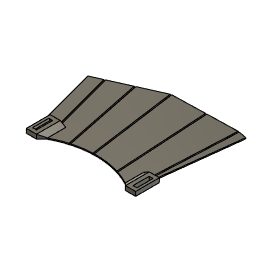
Base-plate (Autodesk Fusion 360 design; units mm, degrees)
Autodesk Fusion 360 part; units mm, degrees
sketch "Sketch1" plane through (0, 0, 0) normal (0, 1, 0) x (1, 0, 0)
  line L0 (-33, 0) -> (52, 0)
  line L1 (-33, 0) -> (-44.6469, 43.4667)
  line L2 (-35.3975, 47.5847) -> (-22.6472, 0)
  line L3 (-18.9537, 54.906) -> (-7.6472, 0)
  line L4 (52, 0) -> (59.5264, 63.5559)
  line L5 (31.5, 0) -> (27.6688, 64.3091)
  line L6 (47.3528, 0) -> (47.3528, -15)
  line L7 (47.3528, -15) -> (-22.6472, -15)
  line L8 (-22.6472, -15) -> (-22.6472, 0)
  line L9 (50.3528, -3.25) -> (52.3528, -3.25)
  line L10 (52.3528, -3.25) -> (52.3528, -15.95)
  line L11 (52.3528, -15.95) -> (50.3528, -15.95)
  line L12 (50.3528, -15.95) -> (50.3528, -3.25)
  line L13 (-27.6472, -3.25) -> (-25.6472, -3.25)
  line L14 (-25.6472, -3.25) -> (-25.6472, -15.95)
  line L15 (-25.6472, -15.95) -> (-27.6472, -15.95)
  line L16 (-27.6472, -15.95) -> (-27.6472, -3.25)
  line L17 (-22.6472, -0.25) -> (-30.6472, -0.25)
  line L18 (-30.6472, -0.25) -> (-30.6472, -18.95)
  line L19 (-30.6472, -18.95) -> (-22.6472, -18.95)
  line L20 (-22.6472, -18.95) -> (-22.6472, -15)
  line L21 (47.3528, -15) -> (47.3528, -18.95)
  line L22 (47.3528, -18.95) -> (55.3528, -18.95)
  line L23 (55.3528, -18.95) -> (55.3528, -0.25)
  line L24 (55.3528, -0.25) -> (47.3528, -0.25)
  line L25 (0.6769, 63.6461) -> (9.5, 0)
  line L26 (49.5, 0) -> (52.6612, 64.9231)
  line L27 (12.3528, -15) -> (10.1055, -68.0076)
  arc A0 (43.4028, -15) -> (-18.6972, -15) centre (12.3528, -72.1043) ccw
  line L28 (-44.6469, 43.4667) -> (-35.3975, 47.5847)
  line L29 (-35.3975, 47.5847) -> (-18.9537, 54.906)
  line L30 (-18.9537, 54.906) -> (0.6769, 63.6461)
  line L31 (0.6769, 63.6461) -> (27.6688, 64.3091)
  line L32 (27.6688, 64.3091) -> (52.6612, 64.9231)
  line L33 (59.5264, 63.5559) -> (52.6612, 64.9231)
  dimension "d1" = 85
  dimension "d2" = 33
  dimension "d4" = 105
  dimension "d5" = 45
  dimension "d12" = 10
  dimension "d15" = 18
  dimension "d19" = 37.5
  dimension "d22" = 7
  dimension "d29" = 15
  dimension "d30" = 2
  dimension "d31" = 12.7
  dimension "d32" = 2
  dimension "d33" = 12.7
  dimension "d34" = 3.25
  dimension "d35" = 3.25
  dimension "d36" = 3
  dimension "d37" = 3
  dimension "d38" = 3
  dimension "d39" = 3
  dimension "d40" = 3
  dimension "d41" = 3
  dimension "d42" = 3
  dimension "d43" = 3
  dimension "d45" = 64
  dimension "d96" = 70
  dimension "d98" = 7
  dimension "d101" = 15
  dimension "d102" = 22
  dimension "d115" = 3.95
  dimension "d116" = 3.95
  dimension "d117" = 21.4884
  dimension "d120" = 27
  dimension "d121" = 25
  dimension "d123" = 99
  dimension "d124" = 18
  dimension "d125" = 65
  dimension "d127" = 65
  constraint coincident L0 L2.end
  constraint parallel L1 L2
  constraint coincident L0 L3.end
  constraint coincident L0 L6.start
  constraint coincident L0 L5.start
  constraint horizontal L0
  constraint perpendicular L0 L6
  constraint perpendicular L6 L7
  constraint perpendicular L0 L8
  constraint horizontal L9
  constraint vertical L10
  constraint horizontal L11
  constraint vertical L12
  constraint horizontal L13
  constraint vertical L14
  constraint horizontal L15
  constraint vertical L16
  constraint coincident L8 L17.start
  constraint perpendicular L8 L17
  constraint perpendicular L17 L18
  constraint perpendicular L18 L19
  constraint perpendicular L7 L20
  constraint perpendicular L7 L21
  constraint perpendicular L21 L22
  constraint perpendicular L7 L23
  constraint coincident L6 L24.end
  constraint perpendicular L6 L24
  constraint coincident origin L0
  constraint midpoint L0 L25.end
  constraint coincident L0 L26.start
  constraint midpoint L7 L27.start
  constraint coincident L7 A0.end
  constraint coincident L7 A0.start
  constraint parallel L28 L29
  constraint parallel L29 L30
  constraint parallel L31 L32
  measures "d1" distance of L0.start L0.end
  measures "d2" distance of origin L0.start
  measures "d4" angle of L0 L1
  measures "d5" distance of L0.start L1.end
  measures "d12" distance of L1 L2
  measures "d15" distance of L2.start L3.start
  measures "d29" distance of L6.start L6.end
  measures "d30" distance of L10.end L11.end
  measures "d31" distance of L9.end L10.end
  measures "d32" distance of L14.end L15.end
  measures "d33" distance of L13.start L15.end
  measures "d34" distance of L0 L13
  measures "d35" distance of L0 L9
  measures "d36" distance of L6 L12
  measures "d37" distance of L8 L14
  measures "d38" distance of L9 L24
  measures "d39" distance of L13 L17
  measures "d40" distance of L16 L18
  measures "d41" distance of L15 L19
  measures "d42" distance of L11 L22
  measures "d43" distance of L10 L23
  measures "d45" distance of L0.end L4.end
  measures "d96" distance of L6 L8
  measures "d98" distance of L4.end L26.end
  measures "d101" distance of L2.end L3.end
  measures "d102" distance of L5.start L25.end
  measures "d115" distance of L7.end A0.end
  measures "d116" distance of L6.end A0.start
  measures "d117" distance of L25.start L3.start
  measures "d120" distance of L25.start L5.end
  measures "d121" distance of L5.end L26.end
  measures "d123" angle of L1 L28
  measures "d124" distance of L5.start L26.start
  measures "d125" radius of A0
  measures "d127" distance of L26.start L26.end
extrude "Extrude1" add sketch "Sketch1" along normal blind 0.35 contours L0 L1 L2 L28 | L0 L2 L3 L29 | L0 L6 L7 L8 A0 | L0 L3 L25 L30 | L8 L17 L18 L19 L20 | L0 L5 L25 L31 | L0 L5 L26 L32 | L0 L4 L26 L33 | L6 L21 L22 L23 L24
sketch "Sketch2" plane through (0, 0.35, 0) normal (0, 1, 0) x (-1, 0, 0)
  line L0 (-47.3528, 15) -> (-47.3528, 18.95)
  line L1 (-47.3528, 18.95) -> (-55.3528, 18.95)
  line L2 (-55.3528, 18.95) -> (-55.3528, 0.25)
  line L3 (-55.3528, 0.25) -> (-47.3528, 0.25)
  line L4 (-47.3528, 0.25) -> (-47.3528, 0)
  line L5 (-47.3528, 0) -> (-52, 0)
  line L6 (-52, 0) -> (-59.5264, -63.5559)
  line L7 (44.6469, -43.4667) -> (33, 0)
  line L8 (33, 0) -> (22.6472, 0)
  line L9 (22.6472, 0) -> (22.6472, 0.25)
  line L10 (22.6472, 0.25) -> (30.6472, 0.25)
  line L11 (30.6472, 0.25) -> (30.6472, 18.95)
  line L12 (30.6472, 18.95) -> (22.6472, 18.95)
  line L13 (22.6472, 18.95) -> (22.6472, 15)
  line L14 (22.6472, 15) -> (18.6972, 15)
  line L15 (22.6472, 0.25) -> (22.6472, 15)
  line L16 (-47.3528, 15) -> (-47.3528, 0.25)
  arc A0 (-43.4028, 15) -> (18.6972, 15) centre (-12.3528, 72.1043) ccw
  line L17 (-43.4028, 15) -> (-47.3528, 15)
  line L18 (-0.6769, -63.6461) -> (44.6469, -43.4667)
  line L19 (-59.5264, -63.5559) -> (-52.6612, -64.9231)
  line L20 (25.6472, 15.95) -> (27.6472, 15.95)
  line L21 (27.6472, 15.95) -> (27.6472, 3.25)
  line L22 (27.6472, 3.25) -> (25.6472, 3.25)
  line L23 (25.6472, 3.25) -> (25.6472, 15.95)
  line L24 (-52.3528, 15.95) -> (-50.3528, 15.95)
  line L25 (-50.3528, 15.95) -> (-50.3528, 3.25)
  line L26 (-50.3528, 3.25) -> (-52.3528, 3.25)
  line L27 (-52.3528, 3.25) -> (-52.3528, 15.95)
  line L28 (-52.6612, -64.9231) -> (-0.6769, -63.6461)
  constraint coincident L9.end L10.start
  constraint coincident L13.end L14.start
  constraint coincident L0.start L16.start
  constraint coincident L3.end L4.start
extrude "Extrude2" add sketch "Sketch2" along normal blind 3 contours L0 L1 L2 L3 L16 | L10 L11 L12 L13 L15
sketch "Sketch3" plane through (0, 0.35, 0) normal (0, 1, 0) x (-1, 0, 0)
  line L0 (-47.3528, 15) -> (-47.3528, 0.25)
  line L1 (-47.3528, 0.25) -> (-47.3528, 0)
  line L2 (-47.3528, 0) -> (-52, 0)
  line L3 (-52, 0) -> (-59.5264, -63.5559)
  line L4 (44.6469, -43.4667) -> (33, 0)
  line L5 (33, 0) -> (22.6472, 0)
  line L6 (22.6472, 0) -> (22.6472, 0.25)
  line L7 (22.6472, 0.25) -> (22.6472, 15)
  line L8 (22.6472, 15) -> (18.6972, 15)
  line L9 (35.3975, -47.5847) -> (22.6472, 0)
  line L10 (-52.6612, -64.9231) -> (-49.5, 0)
  line L11 (18.9537, -54.906) -> (7.6472, 0)
  line L12 (-0.6769, -63.6461) -> (-9.5, 0)
  line L13 (-27.6688, -64.3091) -> (-31.5, 0)
  line L14 (19.4213, -54.6978) -> (5.0689, 15)
  line L15 (18.4861, -55.1142) -> (4.0479, 15)
  line L16 (35.86, -47.3788) -> (23.1649, 0)
  line L17 (34.9351, -47.7906) -> (22.1296, 0)
  line L18 (-0.2015, -63.4344) -> (-11.0746, 15)
  line L19 (-1.18, -63.6585) -> (-12.0842, 15)
  line L20 (-27.1686, -64.2969) -> (-31.8927, 15)
  line L21 (-28.1689, -64.3214) -> (-32.8945, 15)
  line L22 (-52.1654, -65.0218) -> (-48.9994, 0)
  line L23 (-53.157, -64.8243) -> (-50.0006, 0)
  line L24 (22.6472, 0) -> (22.1296, 0)
  line L25 (-52, 0) -> (33, 0)
  arc A0 (-43.4028, 15) -> (18.6972, 15) centre (-12.3528, 72.1043) ccw
  line L26 (-43.4028, 15) -> (-47.3528, 15)
  line L27 (-59.5264, -63.5559) -> (-52.6612, -64.9231)
  line L28 (-0.6769, -63.6461) -> (44.6469, -43.4667)
  line L29 (-52.6612, -64.9231) -> (-0.6769, -63.6461)
  dimension "d61" = 10
  dimension "d62" = 18
  dimension "d63" = 25
  dimension "d74" = 0.5
  dimension "d75" = 0.5
  dimension "d76" = 0.5
  dimension "d77" = 0.5
  dimension "d78" = 0.5
  dimension "d79" = 0.5
  dimension "d80" = 0.5
  dimension "d81" = 0.5
  dimension "d82" = 0.5
  dimension "d83" = 0.5
  dimension "d106" = 7
  dimension "d108" = 15
  dimension "d109" = 22
  dimension "d111" = 18
  constraint coincident L5 L6.start
  constraint coincident L5 L16.end
  constraint horizontal L24
  constraint coincident L2 L23.end
  constraint coincident L2.end L3.start
  constraint coincident L4.end L5.start
  constraint coincident L10.end L25
  constraint coincident L22.end L25
  constraint coincident L25 L11.end
  constraint coincident L25 L12.end
  constraint coincident L25 L13.end
  constraint coincident L8 L14.end
  constraint coincident L8 L15.end
  constraint coincident L8 L18.end
  constraint coincident L8 L19.end
  constraint coincident L8 L21.end
  constraint coincident L8 L20.end
  constraint coincident L10.start L27
  constraint coincident L22.start L27
  constraint coincident L23.start L27
  constraint midpoint L25 L12.end
  constraint coincident L13.start L29
  constraint coincident L21.start L29
  constraint coincident L20.start L29
  constraint coincident L12.start L28.start
  constraint coincident L19.start L29
  constraint coincident L18.start L28
  measures "d61" distance of L4 L9
  measures "d62" distance of L9.start L11.start
  measures "d63" distance of L10.start L13.start
  measures "d74" distance of L10 L23
  measures "d75" distance of L10 L22
  measures "d76" distance of L13 L21
  measures "d77" distance of L13 L20
  measures "d78" distance of L12 L19
  measures "d79" distance of L12 L18
  measures "d80" distance of L11 L15
  measures "d81" distance of L11 L14
  measures "d82" distance of L9 L17
  measures "d83" distance of L9 L16
  measures "d106" distance of L3.end L10.start
  measures "d108" distance of L5.end L11.end
  measures "d109" distance of L12.end L13.end
  measures "d111" distance of L10.end L13.end
extrude "Extrude3" add sketch "Sketch3" along normal blind 0.5 contours L0 L1 L21 L25 A0 L26 | L2 L21 L22 L25 L29 | L19 L20 L25 A0 | L19 L20 L25 L29 | L2 L3 L23 L25 L27 | L15 L18 L25 A0 | L15 L18 L25 L28 | L6 L7 L8 L14 L24 L25 A0 | L14 L17 L25 L28 | L4 L5 L16 L25 L28
chamfer "Chamfer2" distance 0.5 angle 45 10 edges at (50.5797, 0.35, -32.4554) (51.5788, 0.35, -32.4122) (30.393, 0.35, -26.9888) (29.3823, 0.35, -27.1394) (6.0858, 0.35, -28.27) (5.0938, 0.35, -28.1435) (-11.832, 0.35, -22.8006) (-12.7814, 0.35, -22.4535) (-29.5124, 0.35, -23.6894) (-28.5323, 0.35, -23.8953)
chamfer "Chamfer3" distance 2.5 distance2 4.375 2 edges at (47.3528, 0.85, 7.625) (-22.6472, 0.85, 7.625) measured on face at (47.3528, 2.5167, 11.4) measured on face at (-22.6472, 2.5167, 11.4)
chamfer "Chamfer4" distance 3.95 angle 45 2 edges at (-22.6472, 1.675, 15) (47.3528, 1.675, 15)
chamfer "Chamfer5" distance 1 angle 45 4 edges at (-27.6472, 3.35, 9.6) (52.3528, 3.35, 9.6) (-27.6472, 0, 9.6) (52.3528, 0, 9.6)
equation "d32 = d30"
equation "d33 = d31"
equation "d35 = d34"
equation "d61 = d12"
equation "d62 = d15"
equation "d63 = d121"
equation "d74 = d75"
equation "d75 = d76"
equation "d76 = d77"
equation "d77 = d78"
equation "d78 = d79"
equation "d79 = d80"
equation "d80 = d81"
equation "d81 = d82"
equation "d82 = d83"
equation "d84 = d83"
equation "d86 = d83"
equation "d106 = d98"
equation "d108 = d101"
equation "d109 = d102"
equation "d111 = d124"
